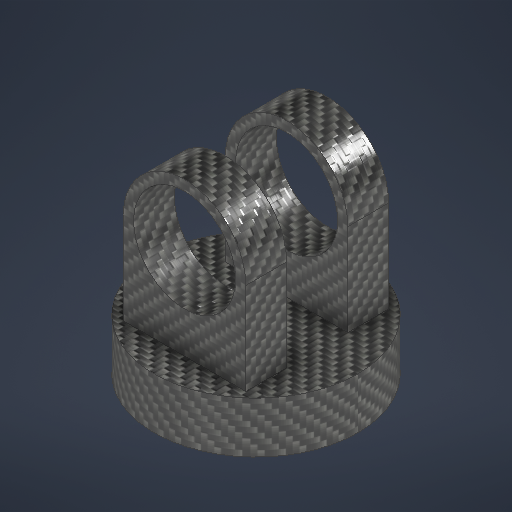
# Autodesk Inventor part: JOINT BASE2
Saved by Autodesk Inventor 2027.1 (Build 311270010, 270A)
## iProperties
Created: 2026-08-28
Part Number: JOINT BASE2
Material: Generic
Document SubType Name: Modeling
Designer: RIDDHIMAN
Density: 1 g/cm^3
Appearance: Default
Author: RIDDHIMAN
Autodesk Inventor part; units mm, degrees
ref_plane "YZ Plane" through (0, 0, 0) normal (1, 0, 0) x (0, 1, 0)
ref_plane "XZ Plane" through (0, 0, 0) normal (0, 1, 0) x (-1, 0, 0)
ref_plane "XY Plane" through (0, 0, 0) normal (0, 0, 1) x (1, 0, 0)
sketch "Sketch1" plane through (0, 0, 0) normal (0, 1, 0) x (-1, 0, 0)
  circle A0 centre (0, 0) radius 50
  dimension "d0" = 100
  constraints: 1 centre point, 1 coincident
  measures "d0" diameter of A0
extrude "Extrusion1" add sketch "Sketch1" along normal blind 25
sketch "Sketch2" plane through (0, 0, 0) normal (0, -1, 0) x (1, 0, 0)
  circle A0 centre (0, 0) radius 25
  dimension "d3" = 50
  constraints: 1 centre point, 1 coincident
  measures "d3" diameter of A0
extrude "Extrusion2" cut sketch "Sketch2" against normal blind 10
sketch "Sketch3" plane through (0, 25, 0) normal (0, 1, 0) x (1, 0, 0)
  line L0 (-30, -35) -> (30, -35)
  line L1 (30, -35) -> (30, 35)
  line L2 (30, 35) -> (-30, 35)
  line L3 (-30, 35) -> (-30, -35)
  line L4 (-30, -35) -> (30, 35) construction
  line L5 (30, -35) -> (-30, 35) construction
  line L6 (-30, -35) -> (30, -35)
  line L7 (30, -35) -> (30, -15)
  line L8 (30, -15) -> (-30, -15)
  line L9 (-30, -15) -> (-30, -35)
  line L10 (-30, 35) -> (30, 35)
  line L11 (30, 35) -> (30, 15)
  line L12 (30, 15) -> (-30, 15)
  line L13 (-30, 15) -> (-30, 35)
  point P0 (0, 0)
  dimension "d6" = 60
  dimension "d7" = 70
  dimension "d8" = 20
  dimension "d9" = 20
  constraints: 28 end point, 6 parallel, 3 horizontal, 3 perpendicular, 2 midpoint, 2 point on line
  measures "d6" distance of L2.end L1.end
  measures "d7" distance of L1.end L0.end
  measures "d8" distance of L7.end L6.end
  measures "d9" distance of L10.end L11.end
extrude "Extrusion3" add sketch "Sketch3" along normal blind 75 contours L3 L8 L1 L0 | L3 L2 L1 L12
sketch "Sketch4" plane through (-30, 25, 35) normal (0, 0, 1) x (1, 0, 0)
  line L0 (60, 0) -> (60, 75) projected
  circle A0 centre (30, 45) radius 30
  line L1 (0, 75) -> (60, 75) projected
  line L2 (60, 0) -> (60, 75) projected
  circle A1 centre (30, 45) radius 25
  line L3 (0, 45) -> (0, 75)
  line L4 (60, 75) -> (60, 45)
  point P0 (30, -25)
  point P1 (30, 75)
  dimension "d12" = 60
  dimension "d13" = 50
  constraints: 4 end point, 2 centre point, 2 point on circle, 2 tangent, 1 coincident, 1 point on line, 1 vertical
  measures "d12" diameter of A0
  measures "d13" diameter of A1
extrude "Extrusion4" cut sketch "Sketch4" against normal blind 100 contours A0 L1 L0 | L3 L1 A0 | A1
body "Solid1"
